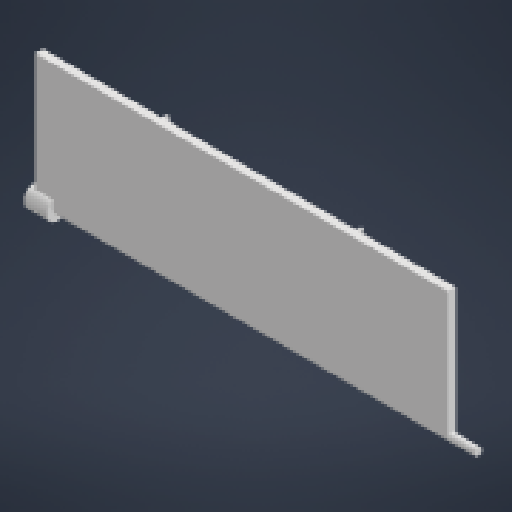
# Autodesk Inventor part: easy doo
Saved by Autodesk Inventor 2026.2 (Build 302298010, 298A)
## iProperties
Created: 2026-03-14
Part Number: easy doo
Material: Generic
Document SubType Name: Modeling
Designer: ba2032
Density: 1 g/cm^3
Appearance: Default
Author: ba2032
Autodesk Inventor part; units mm, degrees
ref_plane "YZ Plane" through (0, 0, 0) normal (1, 0, 0) x (0, 1, 0)
ref_plane "XZ Plane" through (0, 0, 0) normal (0, 1, 0) x (-1, 0, 0)
ref_plane "XY Plane" through (0, 0, 0) normal (0, 0, 1) x (1, 0, 0)
sketch "Sketch1" plane through (0, 0, 0) normal (0, 0, 1) x (1, 0, 0)
  point P0 (0, 0)
sketch "Sketch2" plane through (0, 0, 0) normal (0, 0, 1) x (1, 0, 0)
  line L0 (0, 0) -> (149, 0)
  line L1 (149, 0) -> (149, 50)
  line L2 (149, 50) -> (0, 50)
  line L3 (0, 50) -> (0, 0)
  dimension "d0" = 149
  dimension "d1" = 50
  constraints: 8 end point, 2 parallel, 1 horizontal, 1 perpendicular
  measures "d0" distance of L2.end L1.end
  measures "d1" distance of L1.end L0.end
extrude "Extrusion1" add sketch "Sketch2" along normal blind 3
fillet "Fillet1" radius 1.5 1 edges at (74.5, 0, 3)
fillet "Fillet2" radius 1.5 1 edges at (74.5, 0, 0)
sketch "Sketch10" plane through (0, 0, 0) normal (0, 0, -1) x (-1, 0, 0)
  line L0 (-149, 50) -> (0, 50) projected
  line L1 (-46, 4) -> (-37.889, 50)
  line L2 (-37.889, 50) -> (-36.9042, 49.8264)
  line L3 (-36.9042, 49.8264) -> (-45.0152, 3.8264)
  line L4 (-45.0152, 3.8264) -> (-46, 4)
  line L5 (-46, 4) -> (0.7096, 4) construction
  point P0 (0, 0)
  dimension "d34" = 80
  dimension "d35" = 1
  constraints: 10 end point, 2 parallel, 1 equal length, 1 horizontal, 1 perpendicular, 1 point on line
  measures "d34" angle of L5 L1
  measures "d35" distance of L1.end L2.end
extrude "Extrusion9" add sketch "Sketch10" along normal blind 2
sketch "Sketch11" plane through (0, 0, 0) normal (0, 0, -1) x (-1, 0, 0)
  line L0 (-149, 50) -> (0, 50) projected
  line L1 (-103, 4) -> (-111.111, 50)
  line L2 (-111.111, 50) -> (-112.0958, 49.8264)
  line L3 (-112.0958, 49.8264) -> (-103.9848, 3.8264)
  line L4 (-103.9848, 3.8264) -> (-103, 4)
  line L5 (-103, 4) -> (-56.2904, 4) construction
  point P0 (0, 0)
  dimension "d38" = 100
  dimension "d39" = 1
  constraints: 10 end point, 2 parallel, 1 equal length, 1 horizontal, 1 perpendicular, 1 point on line
  measures "d38" angle of L5 L1
  measures "d39" distance of L2.end L1.end
extrude "Extrusion10" add sketch "Sketch11" along normal blind 2
sketch "Sketch12" plane through (0, 50, 0) normal (-1, 0, 0) x (0, 0, 1)
  circle A0 centre (1.5, -48.5) radius 3
  circle A1 centre (1.5, -48.5) radius 4
  point P0 (0, -50)
  dimension "d43" = 6
  dimension "d49" = 8
  constraints: 2 centre point
  measures "d43" diameter of A0
  measures "d49" diameter of A1
extrude "Extrusion11" add sketch "Sketch12" along normal blind 10 contours A0 | A1
sketch "Sketch13" plane through (149, 50, 3) normal (1, 0, 0) x (0, 0, -1)
  arc A0 (0, -48.5) -> (3, -48.5) centre (1.5, -48.5) ccw projected
  circle A1 centre (1.5, -48.5) radius 1.5
  point P0 (3, -50)
  dimension "d46" = 3
  constraints: 1 centre point, 1 coincident
  measures "d46" diameter of A1
extrude "Extrusion12" add sketch "Sketch13" along normal blind 10
sketch "Sketch15" plane through (0, 50, 0) normal (1, 0, 0) x (0, 0, -1)
  point P0 (0, -50)
sketch "Sketch17" plane through (0, 50, 0) normal (-1, 0, 0) x (0, 0, 1)
  line L0 (3, 0) -> (3, -44.7919) projected
  arc A0 (0, -48.5) -> (3, -48.5) centre (1.5, -48.5) ccw projected
  line L1 (3, 0) -> (3, -48.5)
  line L2 (3, -48.5) -> (0, -48.5)
  line L3 (0, -48.5) -> (0, 0)
  line L4 (0, 0) -> (3, 0)
  point P0 (0, -50)
  constraints: 8 end point, 2 parallel, 1 perpendicular, 1 tangent, 1 vertical
extrude "Extrusion15" add sketch "Sketch17" along normal blind 8 contours L0 L1 L2 L3 L4
sketch "Sketch19" plane through (-10, 1.5, 1.5) normal (-1, 0, 0) x (0, 0, 1)
  circle A0 centre (0, 0) radius 3
  point P0 (-1.5, -1.5)
  dimension "d60" = 6
  constraints: 1 centre point
  measures "d60" diameter of A0
extrude "Extrusion17" cut sketch "Sketch19" against normal blind 8
sketch "Sketch22" plane through (0, 50, 0) normal (1, 0, 0) x (0, 0, -1)
  circle A0 centre (-1.5, -48.5) radius 3 projected
  circle A1 centre (-1.5, -48.5) radius 4
  point P0 (0, -50)
  constraints: 1 centre point, 1 coincident
extrude "Extrusion18" cut sketch "Sketch22" against normal blind 1
sketch "Sketch23" plane through (0, 50, 0) normal (1, 0, 0) x (0, 0, -1)
  circle A0 centre (-1.5, -48.5) radius 1.5 projected
  circle A1 centre (-1.5, -48.5) radius 3
  point P0 (0, -50)
  constraints: 1 centre point, 1 coincident
extrude "Extrusion19" cut sketch "Sketch23" against normal blind 1
sketch "Sketch24" plane through (0, 50, 0) normal (-1, 0, 0) x (0, 0, 1)
  line L0 (3, -44.7919) -> (3, -48.5) projected
  line L1 (0, -44.7919) -> (0, -48.5) projected
  line L2 (3, -44.7919) -> (0, -44.7919)
  line L3 (0, -44.7919) -> (0, -48.5)
  line L4 (0, -48.5) -> (3, -48.5)
  line L5 (3, -48.5) -> (3, -44.7919)
  point P0 (0, -50)
  constraints: 8 end point, 2 parallel, 1 horizontal, 1 perpendicular
extrude "Extrusion20" add sketch "Sketch24" along normal blind 2
body "Solid1"
